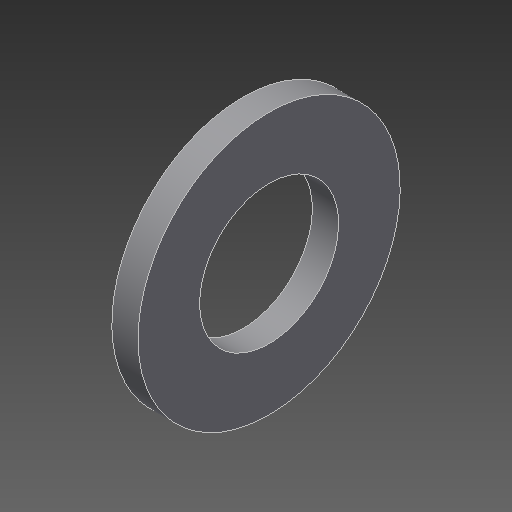
# Autodesk Inventor part: PWF5
Saved by Autodesk Inventor 2021.1 (Build 251245010, 245A)
## iProperties
Created: 2010-03-07
Part Number: PWF5
Catalog Web Link: www.cadenas.de
Document SubType Name: Modeling
Density: 1 g/cm^3
Material: MISUMI
Appearance: 既定
Category: PARTsolutions
NB: PWF5
NN: PWF, SPWF
NT: Flat Washers
NBSYN: $PN.
LINA: PWF5
PN: PWF5
ST: Trivalent Chromate Plating
NO: 5
DD: 5.3
D: 10.0
D1: 10.0
D2: 10.0
TT: 1.0
M1: 5.000
KT: DUMMY
PSOL_IDENT_0: {\\10.0.0.149\dplatte\cadenas\23d-libs\misumi\metric\27_screws_nuts\pwf.prj},156 {VTYP=3D},{NB=PWF5}
PSOL_IDENT_1: ,{LINA=PWF5},{NN=PWF, SPWF},{DATE=27.11.2009 13:53:07},{GEOMDATE=07.07.2009 11:56:00},{VERSION=},{LI
PSOL_IDENT_2: NEID=40},{LINESUBID=-1},{WBVAR=MAT}  {NB=PWF5},{LINA=PWF5},{KT=DUMMY},{PN=PWF5},{MAT=},{ST=Trivalent
PSOL_IDENT_3: Chromate Plating},{NO=5},{DD=5.3},{D=10.0},{D1=10.0},{D2=10.0},{TT=1.0},{M1=5.000}
Title: 平座金
Comments: Flat Washers
Autodesk Inventor part; units mm, degrees
sketch "Sketch_1" plane through (0, 0, 0) normal (0, 0, 1) x (1, 0, 0)
  line L0 (0.5, 0) -> (-0.5, 0)
  line L1 (-0.5, 2.65) -> (0.5, 2.65)
  line L2 (0.5, 2.65) -> (0.5, 5)
  line L3 (0.5, 5) -> (-0.5, 5)
  line L4 (-0.5, 5) -> (-0.5, 2.65)
  constraints: 10 end point
revolve "Revolution1" add sketch "Sketch_1" angle 360 about axis through (0.5, 0, 0) along (1, 0, 0)
ref_plane "plain_washer_to_bolt_XY" through (0, 0, 0) normal (1, 0, 0) x (0, 0, -1)
ref_plane "plain_washer_to_bolt_YZ" through (0, 0, 0) normal (0, 0, -1) x (0, 1, 0)
ref_plane "plain_washer_to_bolt_ZX" through (0, 0, 0) normal (0, 1, 0) x (1, 0, 0)
